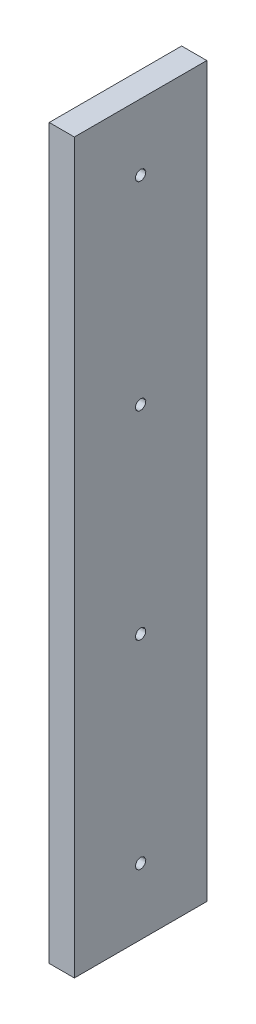
# Autodesk Inventor part: G
Saved by Autodesk Inventor 2024 (Build 280153000, 153)
## iProperties
Created: 2024-03-20
Part Number: G
Material: Generic
Document SubType Name: Modeling
Designer: marco
Density: 1 g/cm^3
Appearance: Wood - Painted White
Author: marco
Autodesk Inventor part; units mm, degrees
ref_plane "YZ Plane" through (0, 0, 0) normal (1, 0, 0) x (0, 1, 0)
ref_plane "XZ Plane" through (0, 0, 0) normal (0, 1, 0) x (-1, 0, 0)
ref_plane "XY Plane" through (0, 0, 0) normal (0, 0, 1) x (1, 0, 0)
sketch "Sketch1" plane through (0, 0, 0) normal (1, 0, 0) x (0, 1, 0)
  line L0 (275, 50) -> (-275, 50)
  line L1 (-275, 50) -> (-275, -50)
  line L2 (-275, -50) -> (275, -50)
  line L3 (275, -50) -> (275, 50)
  circle A0 centre (225, 0) radius 4
  circle A1 centre (75, 0) radius 4
  circle A2 centre (-75, 0) radius 4
  circle A3 centre (-225, 0) radius 4
  point P0 (275, 0)
  point P1 (-275, 0)
  dimension "d0" = 550
  dimension "d1" = 100
  dimension "d7" = 8
  dimension "d8" = 8
  dimension "d9" = 8
  dimension "d10" = 8
  dimension "d11" = 150
  dimension "d12" = 50
  dimension "d13" = 150
  dimension "d14" = 150
  dimension "d15" = 50
  constraints: 8 end point, 4 centre point, 2 midpoint, 2 parallel, 1 horizontal, 1 perpendicular
  measures "d0" distance of L2.end L1.end
  measures "d1" distance of L1.end L0.end
  measures "d7" diameter of A0
  measures "d8" diameter of A1
  measures "d9" diameter of A2
  measures "d10" diameter of A3
  measures "d11" distance of A1.centre A0.centre
  measures "d12" distance of point (275, 0) A0.centre
  measures "d13" distance of A1.centre A2.centre
  measures "d14" distance of A3.centre A2.centre
  measures "d15" distance of point (-275, 0) A3.centre
extrude "Extrusion1" add sketch "Sketch1" along normal mid plane 19
body "Solid1"
